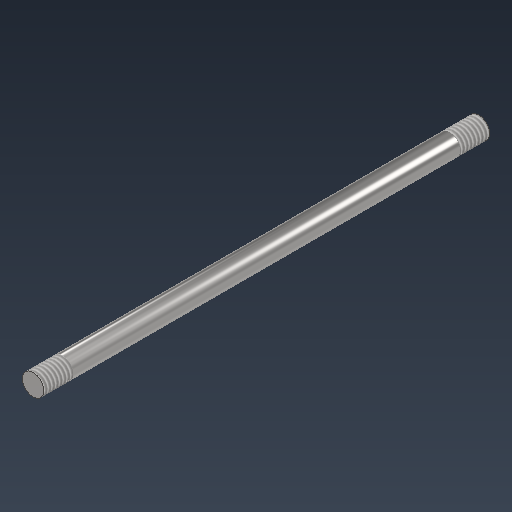
# Autodesk Inventor part: wałek-blatu
Saved by Autodesk Inventor 2026.1 (Build 301233020, 233B)
## iProperties
Created: 2025-11-09
Part Number: wałek-blatu
Material: Stainless Steel
Document SubType Name: Modeling
Designer: Jan
Density: 8 g/cm^3
Appearance: Semi-Polished
Author: Jan
Autodesk Inventor part; units mm, degrees
ref_plane "YZ Plane" through (0, 0, 0) normal (1, 0, 0) x (0, 1, 0)
ref_plane "XZ Plane" through (0, 0, 0) normal (0, 1, 0) x (-1, 0, 0)
ref_plane "XY Plane" through (0, 0, 0) normal (0, 0, 1) x (1, 0, 0)
sketch "Sketch1" plane through (0, 0, 0) normal (0, 0, 1) x (1, 0, 0)
  circle A0 centre (0, 0) radius 2
  dimension "d0" = 4
  constraints: 1 centre point, 1 coincident
  measures "d0" diameter of A0
extrude "Extrusion1" add sketch "Sketch1" along normal blind 83
thread "Thread1" size "M4x0.7" class "6g" standard "ISO Metric profile" length 5.5
thread "Thread2" size "M4x0.7" class "6g" standard "ISO Metric profile" length 5.5
body "Solid1"
